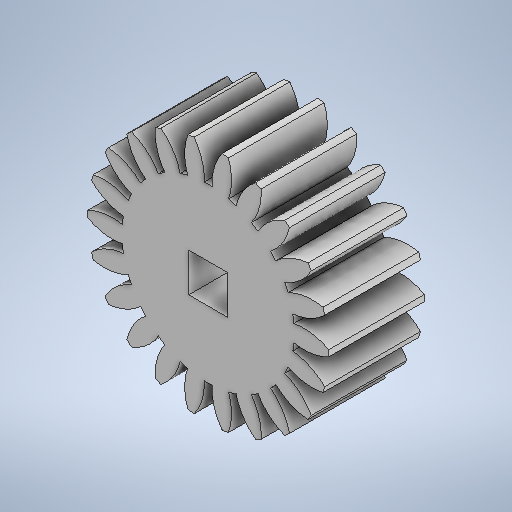
# Autodesk Inventor part: Pinion Gear FV
Saved by Autodesk Inventor 2025.4 (Build 294407000, 407)
## iProperties
Created: 2026-05-10
Part Number: Pinion Gear FV
Material: Generic
Document SubType Name: Modeling
Designer: lenovo
Density: 1 g/cm^3
Appearance: Default
Author: lenovo
Autodesk Inventor part; units mm, degrees
ref_plane "YZ Plane" through (0, 0, 0) normal (1, 0, 0) x (0, 1, 0)
ref_plane "XZ Plane" through (0, 0, 0) normal (0, 1, 0) x (-1, 0, 0)
ref_plane "XY Plane" through (0, 0, 0) normal (0, 0, 1) x (1, 0, 0)
sketch "Sketch1" plane through (0, 0, 0) normal (0, 0, 1) x (1, 0, 0)
  circle A0 centre (0, 0) radius 12.5
  circle A1 centre (0, 0) radius 9
  line L0 (-12.5, 0) -> (12.5, 0)
  line L1 (-2.025, -2.025) -> (2.025, -2.025)
  line L2 (2.025, -2.025) -> (2.025, 2.025)
  line L3 (2.025, 2.025) -> (-2.025, 2.025)
  line L4 (-2.025, 2.025) -> (-2.025, -2.025)
  line L5 (-2.025, -2.025) -> (2.025, 2.025) construction
  line L6 (2.025, -2.025) -> (-2.025, 2.025) construction
  dimension "d0" = 25
  dimension "d1" = 18
  dimension "d7" = 4.05
  constraints: 14 end point, 4 coincident, 3 midpoint, 2 centre point, 2 horizontal, 2 parallel, 2 perpendicular, 2 point on circle
  measures "d0" diameter of A0
  measures "d1" diameter of A1
  measures "d7" distance of L3.end L2.end
extrude "Extrusion1" add sketch "Sketch1" along normal blind 10 contours L0 L2 L3 L4 A1 | A1 L0 L4 L1 L2
sketch "Sketch2" plane through (0, 0, 10) normal (0, 0, 1) x (1, 0, 0)
  line L0 (0, 0) -> (9, 0)
  circle A0 centre (0, 0) radius 9 projected
  circle A1 centre (0, 0) radius 12.6
  arc A2 (12.5958, 0.325) -> (8.9574, 0.875) centre (10.0019, -4.5249) ccw
  arc A3 (8.9574, -0.875) -> (12.5958, -0.325) centre (10.0019, 4.5249) ccw
  point P0 (8.9574, -0.875)
  point P1 (12.5958, -0.325)
  dimension "d17" = 25.2
  dimension "d26" = 0.65
  dimension "d27" = 1.75
  dimension "d28" = 5.5
  constraints: 6 point on circle, 3 symmetric about line, 2 centre point, 2 end point, 1 coincident, 1 horizontal, 4 other
  measures "d26" distance of A2.start A3.end
  measures "d27" diameter of A3.start L0
  measures "d28" radius of A2
extrude "Extrusion2" add sketch "Sketch2" against normal blind 10 contours A0 A2 A1 A3 picked at (10.613, 0.2616)
pattern_circular "Circular Pattern1" count 22 over 360 about axis through (0, 0, -10) along (0, 0, 1) of "Extrusion2"
body "Solid1"
